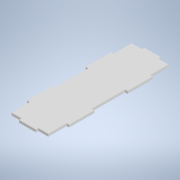
# Autodesk Inventor part: ShortSide
Saved by Autodesk Inventor 2020.3 (Build 243373000, 373)
## iProperties
Created: 2020-08-22
Part Number: ShortSide
Material: Generic
Document SubType Name: Modeling
Designer: Scott Hanson
Density: 1 g/cm^3
Appearance: Default
Author: Scott Hanson
Autodesk Inventor part; units mm, degrees
ref_plane "YZ Plane" through (0, 0, 0) normal (1, 0, 0) x (0, 1, 0)
ref_plane "XZ Plane" through (0, 0, 0) normal (0, 1, 0) x (-1, 0, 0)
ref_plane "XY Plane" through (0, 0, 0) normal (0, 0, 1) x (1, 0, 0)
sketch "Sketch1" plane through (0, 0, 0) normal (0, 1, 0) x (-1, 0, 0)
  line L0 (0, 0) -> (-50, 0)
  line L1 (-50, 0) -> (-50, -150)
  line L2 (-50, -150) -> (0, -150)
  line L3 (0, -150) -> (0, 0)
  dimension "d0" = 150
  dimension "d1" = 50
  constraints: 8 end point, 2 parallel, 1 horizontal, 1 perpendicular
  measures "d0" distance of L2.end L0.start
  measures "d1" distance of L0.start L0.end
extrude "Base" add sketch "Sketch1" along normal blind 3
sketch "Sketch2" plane through (0, 3, 0) normal (0, 1, 0) x (1, 0, 0)
  line L0 (0, 0) -> (50, 0) projected
  line L1 (50, 150) -> (0, 150) projected
  line L2 (0, 0) -> (3, 0)
  line L3 (3, 150) -> (0, 150)
  line L4 (0, 150) -> (0, 0)
  line L5 (0, 150) -> (0, 0) projected
  line L6 (0, 0) -> (3, 0)
  line L7 (3, 0) -> (3, 25)
  line L8 (3, 25) -> (0, 25)
  line L9 (0, 25) -> (0, 0)
  line L10 (0, 150) -> (3, 150)
  line L11 (3, 150) -> (3, 125)
  line L12 (3, 125) -> (0, 125)
  line L13 (0, 125) -> (0, 150)
  line L14 (0, 55) -> (3, 55)
  line L15 (3, 55) -> (3, 95)
  line L16 (3, 95) -> (0, 95)
  line L17 (0, 95) -> (0, 55)
  line L18 (25, 0) -> (25, 150) construction
  line L19 (50, 0) -> (47, 0)
  line L20 (47, 150) -> (50, 150)
  line L21 (50, 150) -> (50, 0)
  line L22 (50, 150) -> (50, 0)
  line L23 (50, 0) -> (47, 0)
  line L24 (47, 0) -> (47, 25)
  line L25 (47, 25) -> (50, 25)
  line L26 (50, 25) -> (50, 0)
  line L27 (50, 150) -> (47, 150)
  line L28 (47, 150) -> (47, 125)
  line L29 (47, 125) -> (50, 125)
  line L30 (50, 125) -> (50, 150)
  line L31 (50, 55) -> (47, 55)
  line L32 (47, 55) -> (47, 95)
  line L33 (47, 95) -> (50, 95)
  line L34 (50, 95) -> (50, 55)
  line L35 (0, 75) -> (50, 75) construction
  line L36 (50, 0) -> (50, 150) projected
  line L37 (15, 0) -> (3, 0)
  line L38 (3, 0) -> (3, 3)
  line L39 (3, 3) -> (15, 3)
  line L40 (15, 3) -> (15, 0)
  line L41 (50, 0) -> (0, 0)
  line L42 (35, 0) -> (47, 0)
  line L43 (47, 3) -> (35, 3)
  line L44 (35, 3) -> (35, 0)
  line L45 (0, 150) -> (50, 150)
  line L46 (25, 150) -> (25, 0) construction
  line L47 (15, 150) -> (3, 150)
  line L48 (3, 147) -> (15, 147)
  line L49 (15, 147) -> (15, 150)
  line L50 (50, 150) -> (0, 150)
  line L51 (47, 147) -> (35, 147)
  line L52 (35, 150) -> (47, 150)
  line L53 (35, 147) -> (35, 150)
  point P0 (0, 25)
  point P1 (0, 125)
  point P2 (3, 150)
  point P3 (0, 150)
  point P4 (0, 95)
  point P5 (0, 55)
  point P6 (50, 125)
  dimension "d10" = 25
  dimension "d11" = 25
  dimension "d12" = 30
  dimension "d13" = 30
  dimension "d14" = 40
  dimension "d15" = 3
  dimension "d21" = 3
  dimension "d22" = 10
  constraints: 100 end point, 34 symmetric about line, 12 point on line, 9 parallel, 5 horizontal, 4 perpendicular, 3 midpoint, 2 other
  measures "d10" distance of L6.end L7.end
  measures "d11" distance of L10.end L11.end
  measures "d12" distance between parallel lines of L14 L8
  measures "d13" distance between parallel lines of L16 L12
  measures "d14" distance of L14.end L15.end
  measures "d15" distance of L7.end L8.end
  measures "d21" distance of L39.end L37.start
  measures "d22" distance from line of L18 L39.end
extrude "Tabs" cut sketch "Sketch2" against normal through all contours L4 L8 L7 L0 | L7 L39 L40 L0 | L4 L16 L15 L14 | L44 L43 L24 L0 | L24 L25 L21 L0 | L4 L1 L11 L12 | L1 L49 L48 L11 | L31 L32 L33 L21 | L1 L28 L51 L53 | L29 L28 L1 L21
equation "\"d11\" = d10"
equation "\"d13\" = d12"
equation "\"d21\" = d15"
body "Solid1"
